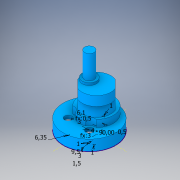
# Autodesk Inventor part: ExcentricShaft
Saved by Autodesk Inventor 2018.3 (Build 223284000, 284)
## iProperties
Created: 2018-07-20
Part Number: ExcentricShaft
Material: Generisch
Document SubType Name: Modeling
Designer: JochenAlt
Density: 1 g/cm^3
Appearance: Vorgabe
Author: JochenAlt
Autodesk Inventor part; units mm, degrees
ref_plane "YZ Plane" through (0, 0, 0) normal (1, 0, 0) x (0, 1, 0)
ref_plane "XZ Plane" through (0, 0, 0) normal (0, 1, 0) x (-1, 0, 0)
ref_plane "XY Plane" through (0, 0, 0) normal (0, 0, 1) x (1, 0, 0)
sketch "Skizze1" plane through (0, 0, 0) normal (0, 0, 1) x (1, 0, 0)
  line L0 (0, 15.7278) -> (0, -15.4546) construction
  line L1 (-15.4546, 0) -> (15.7278, 0) construction
  circle A0 centre (0, 0) radius 2
  arc A1 (0.7505, -5.6701) -> (8.6701, 2.2495) centre (3, 0) ccw
  line L2 (0, 3) -> (0, 0) construction
  line L3 (0, 0) -> (3, 0) construction
  arc A2 (-2.2495, -2.6701) -> (5.6701, 5.2495) centre (0, 3) ccw
  arc A3 (5.2495, 5.6701) -> (-2.6701, -2.2495) centre (3, 0) ccw
  line L4 (0, 0) -> (3, 0) construction
  circle A4 centre (0, 0) radius 9.5
  circle A5 centre (0, 0) radius 11
  circle A6 centre (0, 0) radius 6.35 construction
  circle A7 centre (4.4901, -4.4901) radius 1.5
  circle A8 centre (-4.4901, -4.4901) radius 1.5
  line L5 (4.4901, -4.4901) -> (0, 0) construction
  line L6 (0, 0) -> (-4.4901, -4.4901) construction
  line L7 (2.2495, 8.6701) -> (8.6701, 2.2495)
  line L8 (-5.6701, 0.7505) -> (0.7505, -5.6701)
  line L9 (4.3134, 7.3134) -> (7.3134, 4.3134) construction
  arc A9 (2.2495, 8.6701) -> (-5.6701, 0.7505) centre (0, 3) ccw
  arc A10 (5.6701, 5.2495) -> (2.2495, 8.6701) centre (0, 3) ccw construction
  arc A11 (8.6701, 2.2495) -> (5.2495, 5.6701) centre (3, 0) ccw construction
  arc A12 (-5.6701, 0.7505) -> (-2.2495, -2.6701) centre (0, 3) ccw construction
  arc A13 (-2.6701, -2.2495) -> (0.7505, -5.6701) centre (3, 0) ccw construction
  line L10 (-4.3134, -1.3134) -> (-1.3134, -4.3134) construction
  circle A14 centre (0, 0) radius 3
  circle A15 centre (0, 3) radius 7.1
  circle A16 centre (4.4901, -4.4901) radius 2.5
  circle A17 centre (-4.4901, -4.4901) radius 2.5
  circle A18 centre (3, 0) radius 7.1
  dimension "d0" = 4
  dimension "d1" = 3
  dimension "d14" = 3
  dimension "d15" = 90
  dimension "d16" = 9.5
  dimension "d17" = 1.5
  dimension "d20" = 6.35
  dimension "d21" = 3
  dimension "d26" = 0.5
  dimension "d27" = 0.5
  dimension "d28" = 6.1
  dimension "d31" = 1
  dimension "d34" = 1
  dimension "d37" = 1
  dimension "d40" = 1
  constraints: 23 point on circle, 19 centre point, 18 end point, 9 tangent, 8 coincident, 8 point on line, 6 concentric, 5 equal radius, 3 perpendicular, 2 collinear, 2 parallel
  measures "d0" diameter of A0
  measures "d1" distance of point (0, 0) L2.start
  measures "d14" distance of L2.end L4.end
  measures "d15" angle of L4 L0
  measures "d16" radius of A4
  measures "d17" radial gap between concentric circles of A5 A4
  measures "d20" radius of A6
  measures "d21" diameter of A7
  measures "d26" distance between parallel lines of L9 L7
  measures "d27" distance between parallel lines of L10 L8
  measures "d28" radius of A9
  measures "d31" radial gap between concentric circles of A14 A0
  measures "d34" radial gap between concentric circles of A15 A9
  measures "d37" radial gap between concentric circles of A16 A7
  measures "d40" radial gap between concentric circles of A18 A1
extrude "Extrusion6" add sketch "Skizze1" along normal blind 3 contours A4 A18 | A15 A4 | A5
extrude "Extrusion7" add sketch "Skizze1" along normal blind 1.5 from surface at 3 contours A0 | L8 A15 A16 A1 | A1 A16 A18 A17 A15 L8 | A16 A15 A1 A7 | A1 A7 A16 A18 | A15 A17 A18 L8 | L8 A2 L7 A15 A16 | A7 A1 | A1 A7 | A16 A15 | A18 A16 | A16 A18 A4 A15 A17 | L8 A3 L7 A2 | A17 A18 A15 | A15 A18 A17 | A15 L7 A1 A16 | A16 A1 L7 A15 A18 A4 | A17 A15 A18 | L7 A18 A15 | L8 A18 L7 A3 | A15 A17 A18 | A17 A15 A4 A18 L7 A9 L8 | A4 A18 | L8 A9 L7 A18 | A15 A4 | A15 A4 A18 | A5 | A8 | A14
extrude "Extrusion8" cut sketch "Skizze1" along normal through all both and the other way through all contours A7 A1 | A1 A7 | A8
extrude "Extrusion11" add sketch "Skizze1" along normal blind 3 from surface at 4.5 contours A0 | A15 A17 A18 L8 | L8 A2 L7 A15 A16 | A16 A15 | L8 A3 L7 A2 | A15 A18 A17 | L7 A18 A15 | L8 A18 L7 A3 | A15 A17 A18 | A17 A15 A4 A18 L7 A9 L8 | L8 A9 L7 A18 | A15 A4 | A14 picked at (-2.6547, -3.1388) picked at (-4.0059, -2.6495)
extrude "Extrusion12" cut sketch "Skizze1" along normal blind 3 from surface at 4.5 contours A16 A15 A1 A7 | A1 A7 A16 A18 | A16 A15 | A18 A16 | A17 A18 A15 | A15 A18 A17 | A17 A15 A18 | A15 A17 A18 | A8
extrude "Extrusion2" add sketch "Skizze1" along normal blind 4 from surface at 7.5 contours A0 | L8 A3 L7 A2 | L8 A18 L7 A3 | L8 A9 L7 A18 | A14
extrude "Extrusion3" add sketch "Skizze1" along normal blind 3 from surface at 11.5 contours A0 | L8 A3 L7 A2 | A14
extrude "Extrusion4" add sketch "Skizze1" along normal blind 4 from surface at 14.5 contours A0 | L8 A15 A16 A1 | A16 A15 A1 A7 | L8 A2 L7 A15 A16 | A7 A1 | A16 A15 | L8 A3 L7 A2 | A15 L7 A1 A16 | A14 picked at (4.6073, -4.8832)
extrude "Extrusion10" add sketch "Skizze1" along normal blind 1 from surface at 18.5 contours A0 | A14
extrude "Extrusion14" add sketch "Skizze1" along normal blind 10 from surface at 19.5 contours A0
equation "\"d14\" = d1"
equation "\"d27\" = d26"
